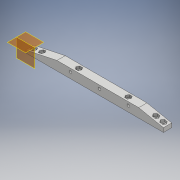
# Autodesk Inventor part: new_wheel_support_v3
Saved by Autodesk Inventor 2017 (Build 210142000, 142)
## iProperties
Created: 2017-08-21
Part Number: new_wheel_support_v3
Material: Generic
Document SubType Name: Modeling
Designer: ndz
Density: 1 g/cm^3
Appearance: Default
Author: ndz
Autodesk Inventor part; units mm, degrees
ref_plane "YZ Plane" through (0, 0, 0) normal (1, 0, 0) x (0, 1, 0)
ref_plane "XZ Plane" through (0, 0, 0) normal (0, 1, 0) x (-1, 0, 0)
ref_plane "XY Plane" through (0, 0, 0) normal (0, 0, 1) x (1, 0, 0)
sketch "Sketch1" plane through (0, 0, 0) normal (0, 0, 1) x (1, 0, 0)
  line L0 (0, 0) -> (167, 0)
  line L1 (167, 0) -> (167, 10)
  line L2 (167, 10) -> (0, 10)
  line L3 (0, 10) -> (0, 0)
  circle A0 centre (59.5, 5) radius 1.6
  circle A1 centre (119.5, 5) radius 1.6
  circle A2 centre (162, 5) radius 1.6
  circle A3 centre (153, 5) radius 1.6
  circle A4 centre (15, 5) radius 1.6
  circle A5 centre (5, 5) radius 1.6
  dimension "d1" = 10
  dimension "d2" = 90
  dimension "d4" = 3.2
  dimension "d6" = 3.2
  dimension "d7" = 3.2
  dimension "d8" = 60
  dimension "d9" = 42.5
  dimension "d26" = 3.2
  dimension "d27" = 33.5
  dimension "d28" = 3.2
  dimension "d29" = 44.5
  dimension "d32" = 15
  dimension "d33" = 5
  dimension "d61" = 3.2
  dimension "d62" = 10
  dimension "d63" = 9
  constraints: 8 end point, 6 centre point, 2 perpendicular, 1 horizontal
  measures "d1" distance of L0.end L1.end
  measures "d2" angle of L1 L0
  measures "d4" diameter of A0
  measures "d6" diameter of A1
  measures "d7" diameter of A2
  measures "d8" distance of A1.centre A0.centre
  measures "d9" distance of A2.centre A1.centre
  measures "d26" diameter of A3
  measures "d27" distance of A3.centre A1.centre
  measures "d28" diameter of A4
  measures "d29" distance of A4.centre A0.centre
  measures "d32" distance from line of L3 A4.centre
  measures "d33" distance from line of L1 A2.centre
  measures "d61" diameter of A5
  measures "d62" distance of A5.centre A4.centre
  measures "d63" distance of A2.centre A3.centre
ref_plane "Work Plane2" through (0, 0, 0) normal (0, -1, 0) x (1, 0, 0)
sketch "Sketch2" plane through (0, 0, 0) normal (0, -1, 0) x (1, 0, 0)
  circle A0 centre (54.5, 7) radius 1.6
  circle A1 centre (124.5, 7) radius 1.6
  circle A2 centre (89.5, 7) radius 1.6
  point P0 (0, 0)
  dimension "d13" = 3.2
  dimension "d15" = 3.2
  dimension "d16" = 70
  dimension "d17" = 3.2
  dimension "d18" = 35
  dimension "d64" = 54.5
  dimension "d65" = 35
  constraints: 3 centre point, 1 horizontal alignment, 1 other
  measures "d13" diameter of A0
  measures "d15" diameter of A1
  measures "d16" distance of A0.centre A1.centre
  measures "d17" diameter of A2
  measures "d18" distance of A0.centre A2.centre
  measures "d64" horizontal distance of point (0, 0) A0.centre
  measures "d65" distance of A1.centre A2.centre
ref_plane "Work Plane1" through (0, 0, 11) normal (0, 0, 1) x (1, 0, 0)
extrude "klocek" add sketch "Sketch1" along normal blind 11
ref_plane "Work Plane3" through (0, 0, 0) normal (0, -1, 0) x (1, 0, 0)
extrude "prowadzenie osi" cut sketch "Sketch2" against normal up to next
ref_plane "Work Plane4" through (0, 0, 0) normal (0, -1, 0) x (1, 0, 0)
sketch "Sketch7" plane through (0, 0, 0) normal (0, -1, 0) x (1, 0, 0)
  line L0 (0, 11) -> (0, 3)
  line L1 (0, 11) -> (167, 11) projected
  line L2 (0, 11) -> (38, 11)
  line L3 (38, 11) -> (0, 3)
  point P0 (0, -1.8333)
  dimension "d86" = 8
  dimension "d87" = 38
  constraints: 6 end point, 1 point on line
  measures "d86" distance of L0.start L0.end
  measures "d87" distance of L0.start L2.end
sketch "Sketch8" plane through (0, 0, 0) normal (0, -1, 0) x (1, 0, 0)
  line L0 (167, 0) -> (167, 11) projected
  line L1 (167, 11) -> (167, 5)
  line L2 (167, 11) -> (0, 11) projected
  line L3 (167, 11) -> (137, 11)
  line L4 (137, 11) -> (167, 5)
  point P0 (0, 0)
  point P1 (40.8333, 11)
  dimension "d80" = 6
  dimension "d81" = 30
  constraints: 6 end point, 2 point on line
  measures "d80" distance of L0.end L1.end
  measures "d81" distance of L0.end L3.end
extrude "przedni skos" cut sketch "Sketch7" against normal up to next
extrude "tylni skos" cut sketch "Sketch8" against normal up to next
ref_plane "Work Plane7" through (0, 0, 11) normal (0, 0, 1) x (1, 0, 0)
sketch "Sketch5" plane through (0, 0, 11) normal (0, 0, 1) x (1, 0, 0)
  line L0 (62.9064, 5) -> (61.2032, 2.05)
  line L1 (61.2032, 2.05) -> (57.7968, 2.05)
  line L2 (57.7968, 2.05) -> (56.0936, 5)
  line L3 (56.0936, 5) -> (57.7968, 7.95)
  line L4 (57.7968, 7.95) -> (61.2032, 7.95)
  line L5 (61.2032, 7.95) -> (62.9064, 5)
  line L6 (122.9064, 5) -> (121.2032, 2.05)
  line L7 (121.2032, 2.05) -> (117.7968, 2.05)
  line L8 (117.7968, 2.05) -> (116.0936, 5)
  line L9 (116.0936, 5) -> (117.7968, 7.95)
  line L10 (117.7968, 7.95) -> (121.2032, 7.95)
  line L11 (121.2032, 7.95) -> (122.9064, 5)
  point P0 (59.5, 5)
  point P1 (119.5, 5)
  point P2 (119.5, 5)
  dimension "d44" = 5.9
  dimension "d45" = 5.9
  constraints: 24 end point, 26 other
  measures "d44" distance between parallel lines of L7 L10
  measures "d45" distance between parallel lines of L1 L4
extrude "hex insert middle" cut sketch "Sketch5" against normal blind 3
ref_plane "Work Plane6" through (0, 0, 11) normal (0, 0, 1) x (1, 0, 0)
sketch "Sketch9" plane through (0, 0, 11) normal (0, 0, 1) x (1, 0, 0)
  line L0 (156.4064, 5) -> (154.7032, 2.05)
  line L1 (154.7032, 2.05) -> (151.2968, 2.05)
  line L2 (151.2968, 2.05) -> (149.5936, 5)
  line L3 (149.5936, 5) -> (151.2968, 7.95)
  line L4 (151.2968, 7.95) -> (154.7032, 7.95)
  line L5 (154.7032, 7.95) -> (156.4064, 5)
  point P0 (0, 0)
  point P1 (153, 5)
  point P2 (153, 5)
  dimension "d51" = 5.9
  constraints: 12 end point, 13 other
  measures "d51" distance between parallel lines of L1 L4
extrude "hex insert rear 1" cut sketch "Sketch9" against normal blind 6
ref_plane "Work Plane5" through (0, 0, 11) normal (0, 0, 1) x (1, 0, 0)
sketch "Sketch10" plane through (0, 0, 11) normal (0, 0, 1) x (1, 0, 0)
  line L0 (160.2968, 7.95) -> (163.7032, 7.95)
  line L1 (163.7032, 7.95) -> (165.4064, 5)
  line L2 (165.4064, 5) -> (163.7032, 2.05)
  line L3 (163.7032, 2.05) -> (160.2968, 2.05)
  line L4 (160.2968, 2.05) -> (158.5936, 5)
  line L5 (158.5936, 5) -> (160.2968, 7.95)
  point P0 (0, 0)
  point P1 (162, 5)
  point P2 (162, 5)
  dimension "d72" = 5.9
  constraints: 12 end point, 1 coincident, 1 horizontal, 13 other
  measures "d72" distance between parallel lines of L0 L3
extrude "hex insert rear 2" cut sketch "Sketch10" against normal blind 7.5
sketch "Sketch13" plane through (0, 0, 11) normal (0, 0, 1) x (1, 0, 0)
  circle A0 centre (5, 5) radius 1.6 projected
  line L0 (8.4064, 5) -> (6.7032, 2.05)
  line L1 (6.7032, 2.05) -> (3.2968, 2.05)
  line L2 (3.2968, 2.05) -> (1.5936, 5)
  line L3 (1.5936, 5) -> (3.2968, 7.95)
  line L4 (3.2968, 7.95) -> (6.7032, 7.95)
  line L5 (6.7032, 7.95) -> (8.4064, 5)
  point P0 (0, 0)
  dimension "d90" = 5.9
  constraints: 12 end point, 1 coincident, 13 other
  measures "d90" distance between parallel lines of L1 L4
extrude "Extrusion18" cut sketch "Sketch13" against normal blind 9
sketch "Sketch16" plane through (0, 0, 11) normal (0, 0, 1) x (1, 0, 0)
  circle A0 centre (15, 5) radius 1.6 projected
  line L0 (18.4064, 5) -> (16.7032, 2.05)
  line L1 (16.7032, 2.05) -> (13.2968, 2.05)
  line L2 (13.2968, 2.05) -> (11.5936, 5)
  line L3 (11.5936, 5) -> (13.2968, 7.95)
  line L4 (13.2968, 7.95) -> (16.7032, 7.95)
  line L5 (16.7032, 7.95) -> (18.4064, 5)
  point P0 (0, 0)
  dimension "d93" = 5.9
  constraints: 12 end point, 1 coincident, 13 other
  measures "d93" distance between parallel lines of L1 L4
extrude "Extrusion19" cut sketch "Sketch16" against normal blind 7.5
body "Solid1"
